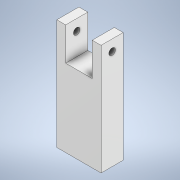
# Autodesk Inventor part: アーム支え
Saved by Autodesk Inventor 2021 (Build 250183000, 183)
## iProperties
Created: 2021-10-07
Part Number: アーム支え
Material: 一般
Document SubType Name: Modeling
Designer: ryusei
Density: 1 g/cm^3
Appearance: 滑らか - 白
Author: ryusei
Autodesk Inventor part; units mm, degrees
ref_plane "YZ Plane" through (0, 0, 0) normal (1, 0, 0) x (0, 1, 0)
ref_plane "XZ Plane" through (0, 0, 0) normal (0, 1, 0) x (-1, 0, 0)
ref_plane "XY Plane" through (0, 0, 0) normal (0, 0, 1) x (1, 0, 0)
sketch "スケッチ1" plane through (0, 0, 0) normal (0, 0, 1) x (1, 0, 0)
  line L0 (0, 0) -> (20, 0)
  line L1 (20, 0) -> (20, 50)
  line L2 (20, 50) -> (0, 50)
  line L3 (0, 50) -> (0, 0)
  dimension "d0" = 20
  dimension "d1" = 50
  constraints: 8 end point, 2 parallel, 1 horizontal, 1 perpendicular
  measures "d0" distance between parallel lines of L1 L3
  measures "d1" distance between parallel lines of L0 L2
extrude "押し出し1" add sketch "スケッチ1" along normal blind 10
sketch "スケッチ2" plane through (0, 0, 10) normal (0, 0, 1) x (1, 0, 0)
  line L0 (20, 50) -> (0, 50) projected
  line L1 (4, 50) -> (16, 50)
  line L2 (16, 50) -> (16, 40)
  line L3 (16, 40) -> (4, 40)
  line L4 (4, 40) -> (4, 50)
  line L5 (0, 50) -> (0, 0) projected
  dimension "d4" = 12
  dimension "d5" = 4
  dimension "d6" = 10
  constraints: 8 end point, 2 parallel, 1 horizontal, 1 perpendicular, 1 point on line
  measures "d4" distance between parallel lines of L2 L4
  measures "d5" distance between parallel lines of L5 L4
  measures "d6" distance between parallel lines of L3 L0
extrude "押し出し2" cut sketch "スケッチ2" against normal blind 10
sketch "スケッチ3" plane through (20, 0, 0) normal (1, 0, 0) x (0, 0, -1)
  line L0 (0, 50) -> (-10, 50) projected
  line L1 (0, 0) -> (0, 50) projected
  point P0 (-5, 45)
  dimension "d9" = 5
  dimension "d10" = 5
  measures "d9" distance from line of L0 point (-5, 45)
  measures "d10" distance from line of L1 point (-5, 45)
hole "穴1" at (20, 45, 5) direction (-1, 0, 0) diameter 3 end through all
sketch "スケッチ4" plane through (0, 0, 0) normal (0, -1, 0) x (1, 0, 0)
  line L0 (0, 0) -> (0, 10) projected
  line L1 (0, 10) -> (20, 10) projected
  line L2 (0, 0) -> (20, 0) projected
  line L3 (20, 0) -> (20, 10) projected
  point P0 (5, 5)
  point P1 (15, 5)
  dimension "d18" = 5
  dimension "d19" = 5
  dimension "d20" = 5
  dimension "d21" = 5
  measures "d18" distance from line of L0 point (5, 5)
  measures "d19" distance from line of L1 point (5, 5)
  measures "d20" distance from line of L2 point (15, 5)
  measures "d21" distance from line of L3 point (15, 5)
hole "穴2" at (5, 0, 5) at (15, 0, 5) direction (0, 1, 0) diameter 2.459 depth 25 tip angle 118 thread size "M3x0.5" class "6H" standard "ISO Metric profile"
sketch "スケッチ5" plane through (0, 0, 10) normal (0, 0, 1) x (1, 0, 0)
  line L0 (4, 40) -> (16, 40) projected
  line L1 (4, 40) -> (16, 40)
  line L2 (16, 40) -> (16, 35)
  line L3 (16, 35) -> (4, 35)
  line L4 (4, 35) -> (4, 40)
  point P0 (0, 0)
  dimension "d29" = 5
  constraints: 8 end point, 2 parallel, 1 horizontal, 1 perpendicular
  measures "d29" distance between parallel lines of L3 L0
extrude "押し出し3" cut sketch "スケッチ5" against normal blind 10
